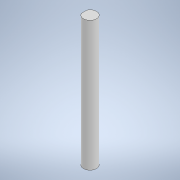
# Autodesk Inventor part: wał_uzębienia
Saved by Autodesk Inventor 2020 (Build 240168000, 168)
## iProperties
Created: 2020-08-10
Part Number: wał_uzębienia
Material: Generic
Document SubType Name: Modeling
Designer: Hesekiel
Density: 1 g/cm^3
Appearance: Default
Author: Hesekiel
Autodesk Inventor part; units mm, degrees
ref_plane "XZ Plane" through (0, 0, 0) normal (0, 1, 0) x (-1, 0, 0)
ref_plane "XY Plane" through (0, 0, 0) normal (0, 0, 1) x (1, 0, 0)
sketch "Sketch1" plane through (0, 0, 0) normal (0, 1, 0) x (-1, 0, 0)
  circle A0 centre (0, 0) radius 5
  dimension "d0" = 10
  constraints: 1 centre point, 1 coincident
  measures "d0" diameter of A0
extrude "Extrusion1" add sketch "Sketch1" along normal blind 100
ref_plane "Work Plane1" through (0, 72.5, 0) normal (0, 1, 0) x (1, 0, 0)
sketch "Sketch2" plane through (0, 72.5, 0) normal (0, 1, 0) x (1, 0, 0)
  circle A0 centre (0, 0) radius 5 projected
ref_plane "Work Plane2" through (-5, 0, 0) normal (1, 0, 0) x (0, 1, 0)
ref_plane "Work Plane3" through (0, 27.5, 0) normal (0, -1, 0) x (1, 0, 0)
sketch "Sketch3" plane through (-5, 0, 0) normal (1, 0, 0) x (0, 1, 0)
  line L0 (27.5, -7) -> (27.5, 7) projected
  line L1 (72.5, 7) -> (72.5, -7) projected
  circle A0 centre (27.5, 0) radius 3
  circle A1 centre (72.5, 0) radius 3
  circle A2 centre (27.5, 0) radius 0.75
  circle A3 centre (72.5, 0) radius 0.75
  line L2 (0, -5) -> (0, 5) projected
  line L3 (27.5, -3) -> (0, -3)
  line L4 (0, -3) -> (0, 3)
  line L5 (0, 3) -> (27.5, 3)
  line L6 (27.5, 3) -> (27.5, -3)
  line L7 (100, -5) -> (100, 5) projected
  line L8 (72.5, -3) -> (100, -3)
  line L9 (100, -3) -> (100, 3)
  line L10 (100, 3) -> (72.5, 3)
  line L11 (72.5, 3) -> (72.5, -3)
  point P0 (0, 0)
  point P1 (72.5, 3)
  point P2 (27.5, 3)
  dimension "d5" = 6
  dimension "d6" = 6
  dimension "d7" = 1.5
  dimension "d8" = 1.5
  constraints: 16 end point, 5 point on line, 4 parallel, 2 centre point, 2 coincident, 2 horizontal, 2 midpoint, 2 perpendicular, 6 other
  measures "d7" diameter of A2
  measures "d8" diameter of A3
extrude "Extrusion2" cut sketch "Sketch3" along normal blind 1 contours A2 L0 | L0 A2 | A3 L1 | L1 A3
extrude "Extrusion3" cut sketch "Sketch3" along normal blind 0.5 contours A0 L0 A2 | L3 L2 L5 A0 | L0 A2 A0 | A1 L1 A3 | L10 L7 L8 A1 | L1 A3 A1
chamfer "Chamfer1" distance 0.5 angle 45 1 edges at (-4.5, 26.75, 0)
chamfer "Chamfer2" distance 0.5 angle 45 1 edges at (-4.5, 71.75, 0)
body "Solid1"
